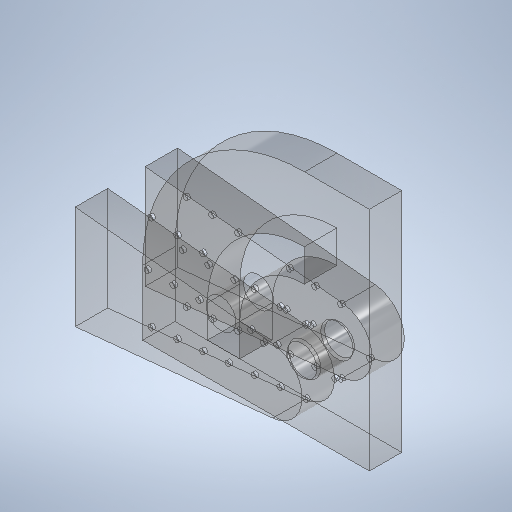
# Autodesk Inventor part: Prueba de soportes mecanismoPruebaPerimetro7
Saved by Autodesk Inventor 2025.2 (Build 292293000, 293)
## iProperties
Created: 2025-03-25
Part Number: Prueba de soportes mecanismoPruebaPerimetro7
Material: PVC, no plastificado
Document SubType Name: Modeling
Designer: braug
Density: 1.29 g/cm^3
Appearance: Agua Burbujas
Author: braug
## iProperties of the stored document Prueba de soportes mecanismo_3DPrint.ipt
Created: 2025-03-25
Part Number: Prueba de soportes mecanismo_3DPrint
Material: Genérico
Document SubType Name: Modeling
Designer: braug
Density: 1 g/cm^3
Appearance: Valor por defecto
Author: braug
Autodesk Inventor part; units mm, degrees
ref_plane "YZ Plane" through (0, 0, 0) normal (1, 0, 0) x (0, 1, 0)
ref_plane "XZ Plane" through (0, 0, 0) normal (0, 1, 0) x (-1, 0, 0)
ref_plane "XY Plane" through (0, 0, 0) normal (0, 0, 1) x (1, 0, 0)
sketch "Boceto1" plane through (0, 0, 0) normal (0, 0, 1) x (1, 0, 0)
  line L0 (-35, 0) -> (15, 0)
  line L1 (-20, 10) -> (-20, 0)
  arc A0 (-10, 20) -> (-20, 10) centre (-10, 10) ccw
  arc A1 (-10, 25) -> (-25, 10) centre (-10, 10) ccw
  line L2 (-25, 10) -> (-25, 0)
  arc A2 (-10, 35) -> (-35, 10) centre (-10, 10) ccw
  line L3 (-35, 10) -> (-35, 0)
  line L4 (-35, 0) -> (-10, 0)
  circle A3 centre (-10, 10) radius 2.5
  line L5 (-10, 20) -> (0, 20)
  line L6 (0, 20) -> (0, 21.1803)
  line L7 (0, 25) -> (-10, 25)
  line L8 (-10, 35) -> (0, 35)
  line L9 (0, 35) -> (0, 25)
  line L10 (0, 20) -> (0, 0)
  line L11 (0, 0) -> (-10, 0)
  line L12 (0, 25) -> (0, 20)
  line L13 (-10, 25) -> (-10, 20)
  line L14 (-20, 5) -> (-25, 5)
  point P0 (0, 0)
  dimension "d0" = 20
  dimension "d1" = 25
  dimension "d2" = 10
  dimension "d3" = 10
  dimension "d4" = 5
  dimension "d6" = 35
  constraints: 30 end point, 7 point on circle, 5 point on line, 4 centre point, 3 coincident, 3 collinear, 3 midpoint, 3 perpendicular, 3 tangent, 2 parallel, 1 horizontal
  measures "d0" distance of L5.start L11.end
  measures "d1" distance of L7.end L11.end
  measures "d2" distance of L3.start L0.start
  measures "d3" distance of L11.end A2.centre
  measures "d4" diameter of A3
  measures "d6" distance of L10.end L8.end
extrude "Extrusión1" add sketch "Boceto1" along normal mid plane 5 contours L3 A2 L8 L9 L7 A1 L2 L0 | L2 L14 L1 L0 | L1 A0 L5 L10 L0 | L7 L12 L6 L5 L13
sketch "Boceto2" plane through (0, 0, 2.5) normal (0, 0, 1) x (1, 0, 0)
  circle A0 centre (-10, 10) radius 2.3
  circle A1 centre (-22.5, 10) radius 2.3
  circle A2 centre (-10, 10) radius 2.5 projected
  point P0 (0, 0)
  dimension "d9" = 4.6
  dimension "d10" = 4.6
  constraints: 2 centre point
  measures "d9" diameter of A0
  measures "d10" diameter of A1
extrude "Extrusión2" add sketch "Boceto2" along normal blind 0.4 and the other way blind 5.4 contours A0 | A1
sketch "Boceto3" plane through (-10, 10, 2.9) normal (0, 0, 1) x (1, 0, 0)
  arc A0 (5, 0) -> (0.4927, 4.9757) centre (0, 0) ccw
  line L0 (-30, 0) -> (-30, 7.9951)
  line L1 (0.4927, 4.9757) -> (-30, 7.9951)
  line L2 (-30, 0) -> (-30, -7.9951)
  line L3 (0.4927, -4.9757) -> (-30, -7.9951)
  arc A1 (0.4927, -4.9757) -> (5, 0) centre (0, 0) ccw
  circle A2 centre (0, 0) radius 2.3 projected
  point P0 (10, -10)
  dimension "d15" = 10
  constraints: 8 end point, 4 point on circle, 2 centre point
  measures "d15" diameter of A0
extrude "Extrusión3" add sketch "Boceto3" along normal blind 5 contours A1 L3 L2 L0 L1 A0 | A2
sketch "Boceto4" plane through (-22.5, 10, -2.9) normal (0, 0, -1) x (-1, 0, 0)
  circle A0 centre (0, 0) radius 2.3 projected
  circle A1 centre (-12.5, 0) radius 2.3 projected
  line L0 (-12.9927, 4.9757) -> (17.5, 7.9951) projected
  arc A2 (-12.9927, 4.9757) -> (-12.9927, -4.9757) centre (-12.5, 0) ccw projected
  line L1 (17.5, -7.9951) -> (-12.9927, -4.9757) projected
  line L2 (17.5, 7.9951) -> (17.5, -7.9951) projected
  point P0 (-22.5, -10)
extrude "Extrusión4" add sketch "Boceto4" along normal blind 5 contours A0 | A1 | L0 L2 L1 A2
sketch "Boceto5" plane through (0, 0, -2.5) normal (0, 0, -1) x (-1, 0, 0)
  arc A0 (9.5073, 14.9757) -> (9.5073, 5.0243) centre (10, 10) ccw construction
  circle A1 centre (5, 10) radius 0.4
  circle A2 centre (9.5073, 14.9757) radius 0.4
  line L0 (9.5073, 14.9757) -> (40, 17.9951) projected
  circle A3 centre (13.4878, 15.3698) radius 0.4
  circle A4 centre (17.4684, 15.764) radius 0.4
  circle A5 centre (21.4489, 16.1581) radius 0.4
  circle A6 centre (25.4294, 16.5523) radius 0.4
  circle A7 centre (29.41, 16.9465) radius 0.4
  circle A8 centre (33.3905, 17.3406) radius 0.4
  line L1 (-2.4318, 10) -> (67.5847, 10) construction
  arc A9 (9.5073, 14.9757) -> (9.5073, 5.0243) centre (10, 10) ccw
  circle A10 centre (9.5073, 5.0243) radius 0.4
  line L2 (9.5073, 5.0243) -> (40, 2.0049)
  circle A11 centre (13.4878, 4.6302) radius 0.4
  circle A12 centre (17.4684, 4.236) radius 0.4
  circle A13 centre (21.4489, 3.8419) radius 0.4
  circle A14 centre (25.4294, 3.4477) radius 0.4
  circle A15 centre (29.41, 3.0535) radius 0.4
  circle A16 centre (33.3905, 2.6594) radius 0.4
  circle A17 centre (10, 10) radius 0.4
  circle A18 centre (14, 10) radius 0.4
  circle A19 centre (18, 10) radius 0.4
  circle A20 centre (22, 10) radius 0.4
  circle A21 centre (26, 10) radius 0.4
  circle A22 centre (30, 10) radius 0.4
  circle A23 centre (34, 10) radius 0.4
  point P0 (0, 0)
  dimension "d45" = 0.8
  dimension "d46" = 0.8
  dimension "d49" = 4
  dimension "d54" = 0.8
  dimension "d57" = 4
  constraints: 23 centre point, 10 symmetric about line, 4 end point, 3 point on circle, 2 horizontal, 33 other
  measures "d45" diameter of A1
  measures "d46" diameter of A2
  measures "d49" distance of A2.centre A3.centre
  measures "d54" diameter of A17
  measures "d57" distance of A17.centre A18.centre
extrude "Extrusión5" add sketch "Boceto5" against normal up to surface (5.4 mm away) contours A1 A9 | A16 L2 | L2 A16 | A15 L2 | L2 A15 | A14 L2 | L2 A14 | A13 L2 | L2 A13 | A12 L2 | L2 A12 | A11 L2 | L2 A11 | A10 L2 A9 | A9 L2 A10 | A8 L0 | L0 A8 | A7 L0 | L0 A7 | A6 L0 | L0 A6 | A4 L0 | L0 A4 | A3 L0 | L0 A3 | A2 L0 A9 | A9 L0 A2 | A9 A1 | A18 | A19 | A21 | A22 | A23
mirror "Simetría1" about plane through (0, 0, 0) normal (0, 0, 1) of "Extrusión5"
